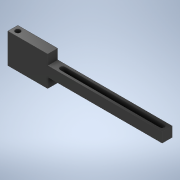
# Autodesk Inventor part: Top Piece
Saved by Autodesk Inventor 2021 (Build 250183000, 183)
## iProperties
Created: 2021-04-03
Part Number: Top Piece
Material: Generic
Document SubType Name: Modeling
Designer: Darek
Density: 1 g/cm^3
Appearance: Default
Mass: 17.7146 g
Surface Area: 99.4978 cm^2
Volume: 17.7146 cm^3
Author: Darek
Autodesk Inventor part; units mm, degrees
ref_plane "YZ Plane" through (0, 0, 0) normal (1, 0, 0) x (0, 1, 0)
ref_plane "XZ Plane" through (0, 0, 0) normal (0, 1, 0) x (-1, 0, 0)
ref_plane "XY Plane" through (0, 0, 0) normal (0, 0, 1) x (1, 0, 0)
sketch "Sketch1" plane through (0, 0, 0) normal (0, 0, 1) x (1, 0, 0)
  line L0 (0, 0) -> (40, 0)
  line L1 (40, 0) -> (40, 30)
  line L2 (40, 30) -> (0, 30)
  line L3 (0, 30) -> (0, 0)
  line L4 (40, 20) -> (155, 20)
  line L5 (155, 20) -> (155, 10)
  line L6 (155, 10) -> (40, 10)
  line L7 (40, 10) -> (40, 20)
  point P0 (40, 10)
  dimension "d0" = 30
  dimension "d1" = 40
  dimension "d2" = 10
  dimension "d3" = 115
  dimension "d4" = 10
  constraints: 16 end point, 4 parallel, 2 horizontal, 2 perpendicular, 1 point on line
  measures "d0" distance between parallel lines of L0 L2
  measures "d1" distance between parallel lines of L1 L3
  measures "d2" distance from line of L0 L5.end
  measures "d3" distance between parallel lines of L1 L5
  measures "d4" distance between parallel lines of L6 L4
extrude "Extrusion1" add sketch "Sketch1" along normal blind 10
sketch "Sketch2" plane through (40, 20, 0) normal (0, 1, 0) x (1, 0, 0)
  circle A0 centre (110, -5) radius 2.5
  circle A1 centre (10, -5) radius 2.5
  line L0 (115, 0) -> (115, -10) projected
  line L1 (115, -10) -> (0, -10) projected
  line L2 (0, 0) -> (0, -10) projected
  line L3 (110, -7.5) -> (10, -7.5)
  line L4 (10, -7.5) -> (10, -2.5)
  line L5 (10, -2.5) -> (110, -2.5)
  line L6 (110, -2.5) -> (110, -7.5)
  point P0 (-40, 0)
  point P1 (110, -2.5)
  point P2 (10, -7.5)
  point P3 (10, -7.5)
  dimension "d8" = 5
  dimension "d12" = 5
  dimension "d9" = 5
  dimension "d10" = 5
  dimension "d11" = 10
  dimension "d14" = 2.5
  dimension "d22" = 100
  dimension "d23" = 5
  constraints: 8 end point, 2 parallel, 1 horizontal, 1 perpendicular, 6 other
  measures "d9" distance from line of L1 point (110, -5)
  measures "d10" distance from line of L1 point (10, -5)
  measures "d11" distance from line of point (10, -5) L2
  measures "d14" distance between parallel lines of L3 L1
  measures "d22" distance of L4.end L5.end
  measures "d23" distance between parallel lines of L3 L5
extrude "Extrusion2" cut sketch "Sketch2" against normal blind 10
sketch "Sketch3" plane through (0, 30, 0) normal (0, 1, 0) x (1, 0, 0)
  circle A0 centre (5, -5) radius 2.5
  line L0 (0, 0) -> (0, -10) projected
  line L1 (40, 0) -> (0, 0) projected
  dimension "d17" = 5
  dimension "d18" = 5
  dimension "d19" = 5
  constraints: 1 centre point
  measures "d17" diameter of A0
  measures "d18" distance from line of A0.centre L0
  measures "d19" distance from line of L1 A0.centre
extrude "Extrusion3" cut sketch "Sketch3" against normal blind 30
body "Solid1"
